镂空抽屉 (Autodesk Fusion 360 design; units mm, degrees)
part number: 2026-05-01-18-35-40-884
Autodesk Fusion 360 part; units mm, degrees
(part 1 of 2)
other "基础网格特征2"
other "修改1"
sketch "草图66" plane through (0, 0, 0) normal (0, 0, 1) x (1, 0, 0)
  line L0 (-100, -100) -> (100, -100)
  line L1 (100, -100) -> (100, 100)
  line L2 (100, 100) -> (-100, 100)
  line L3 (-100, 100) -> (-100, -100)
extrude "ex_drawer_body" add sketch "草图66" along normal blind 50
fillet "fillet_drawer_corners" radius 10 4 edges at (-100, 100, 25) (100, 100, 25) (100, -100, 25) (-100, -100, 25)
shell "shell_drawer" thickness 2 removed faces 1 at (30, -33.3333, 50)
sketch "草图68" plane through (0, -100, 0) normal (0, -1, 0) x (1, 0, 0)
  line L0 (-90, 50) -> (-90, 0)
  line L1 (-90, 0) -> (90, 0)
  line L2 (90, 0) -> (90, 50)
  line L3 (90, 50) -> (-90, 50)
  line L4 (-32.5, 44) -> (32.5, 44)
  line L5 (32.5, 29) -> (-32.5, 29)
  arc A0 (32.5, 29) -> (32.5, 44) centre (32.5, 36.5) ccw
  arc A1 (-32.5, 44) -> (-32.5, 29) centre (-32.5, 36.5) ccw
extrude "cut_grip_drawer" cut sketch "草图68" against normal blind 3 contours L4 L5 A0 A1
sketch "草图69" plane through (-100, 0, 0) normal (-1, 0, 0) x (0, -1, 0)
  line L0 (90, 0) -> (90, 50)
  line L1 (90, 50) -> (-90, 50)
  line L2 (-90, 50) -> (-90, 0)
  line L3 (-90, 0) -> (90, 0)
  line L4 (-81, 14) -> (-85.3301, 11.5)
  line L5 (-85.3301, 11.5) -> (-85.3301, 6.5)
  line L6 (-85.3301, 6.5) -> (-81, 4)
  line L7 (-81, 4) -> (-76.6699, 6.5)
  line L8 (-76.6699, 6.5) -> (-76.6699, 11.5)
  line L9 (-76.6699, 11.5) -> (-81, 14)
  line L10 (-70.3397, 14) -> (-74.6699, 11.5)
  line L11 (-74.6699, 11.5) -> (-74.6699, 6.5)
  line L12 (-74.6699, 6.5) -> (-70.3397, 4)
  line L13 (-70.3397, 4) -> (-66.0096, 6.5)
  line L14 (-66.0096, 6.5) -> (-66.0096, 11.5)
  line L15 (-66.0096, 11.5) -> (-70.3397, 14)
  line L16 (-59.6795, 14) -> (-64.0096, 11.5)
  line L17 (-64.0096, 11.5) -> (-64.0096, 6.5)
  line L18 (-64.0096, 6.5) -> (-59.6795, 4)
  line L19 (-59.6795, 4) -> (-55.3494, 6.5)
  line L20 (-55.3494, 6.5) -> (-55.3494, 11.5)
  line L21 (-55.3494, 11.5) -> (-59.6795, 14)
  line L22 (-49.0192, 14) -> (-53.3494, 11.5)
  line L23 (-53.3494, 11.5) -> (-53.3494, 6.5)
  line L24 (-53.3494, 6.5) -> (-49.0192, 4)
  line L25 (-49.0192, 4) -> (-44.6891, 6.5)
  line L26 (-44.6891, 6.5) -> (-44.6891, 11.5)
  line L27 (-44.6891, 11.5) -> (-49.0192, 14)
  line L28 (-38.359, 14) -> (-42.6891, 11.5)
  line L29 (-42.6891, 11.5) -> (-42.6891, 6.5)
  line L30 (-42.6891, 6.5) -> (-38.359, 4)
  line L31 (-38.359, 4) -> (-34.0289, 6.5)
  line L32 (-34.0289, 6.5) -> (-34.0289, 11.5)
  line L33 (-34.0289, 11.5) -> (-38.359, 14)
  line L34 (-27.6987, 14) -> (-32.0289, 11.5)
  line L35 (-32.0289, 11.5) -> (-32.0289, 6.5)
  line L36 (-32.0289, 6.5) -> (-27.6987, 4)
  line L37 (-27.6987, 4) -> (-23.3686, 6.5)
  line L38 (-23.3686, 6.5) -> (-23.3686, 11.5)
  line L39 (-23.3686, 11.5) -> (-27.6987, 14)
  line L40 (-17.0385, 14) -> (-21.3686, 11.5)
  line L41 (-21.3686, 11.5) -> (-21.3686, 6.5)
  line L42 (-21.3686, 6.5) -> (-17.0385, 4)
  line L43 (-17.0385, 4) -> (-12.7083, 6.5)
  line L44 (-12.7083, 6.5) -> (-12.7083, 11.5)
  line L45 (-12.7083, 11.5) -> (-17.0385, 14)
  line L46 (-6.3782, 14) -> (-10.7083, 11.5)
  line L47 (-10.7083, 11.5) -> (-10.7083, 6.5)
  line L48 (-10.7083, 6.5) -> (-6.3782, 4)
  line L49 (-6.3782, 4) -> (-2.0481, 6.5)
  line L50 (-2.0481, 6.5) -> (-2.0481, 11.5)
  line L51 (-2.0481, 11.5) -> (-6.3782, 14)
  line L52 (4.282, 14) -> (-0.0481, 11.5)
  line L53 (-0.0481, 11.5) -> (-0.0481, 6.5)
  line L54 (-0.0481, 6.5) -> (4.282, 4)
  line L55 (4.282, 4) -> (8.6122, 6.5)
  line L56 (8.6122, 6.5) -> (8.6122, 11.5)
  line L57 (8.6122, 11.5) -> (4.282, 14)
  line L58 (14.9423, 14) -> (10.6122, 11.5)
  line L59 (10.6122, 11.5) -> (10.6122, 6.5)
  line L60 (10.6122, 6.5) -> (14.9423, 4)
  line L61 (14.9423, 4) -> (19.2724, 6.5)
  line L62 (19.2724, 6.5) -> (19.2724, 11.5)
  line L63 (19.2724, 11.5) -> (14.9423, 14)
  line L64 (25.6025, 14) -> (21.2724, 11.5)
  line L65 (21.2724, 11.5) -> (21.2724, 6.5)
  line L66 (21.2724, 6.5) -> (25.6025, 4)
  line L67 (25.6025, 4) -> (29.9327, 6.5)
  line L68 (29.9327, 6.5) -> (29.9327, 11.5)
  line L69 (29.9327, 11.5) -> (25.6025, 14)
  line L70 (36.2628, 14) -> (31.9327, 11.5)
  line L71 (31.9327, 11.5) -> (31.9327, 6.5)
  line L72 (31.9327, 6.5) -> (36.2628, 4)
  line L73 (36.2628, 4) -> (40.5929, 6.5)
  line L74 (40.5929, 6.5) -> (40.5929, 11.5)
  line L75 (40.5929, 11.5) -> (36.2628, 14)
  line L76 (46.923, 14) -> (42.5929, 11.5)
  line L77 (42.5929, 11.5) -> (42.5929, 6.5)
  line L78 (42.5929, 6.5) -> (46.923, 4)
  line L79 (46.923, 4) -> (51.2532, 6.5)
  line L80 (51.2532, 6.5) -> (51.2532, 11.5)
  line L81 (51.2532, 11.5) -> (46.923, 14)
  line L82 (57.5833, 14) -> (53.2532, 11.5)
  line L83 (53.2532, 11.5) -> (53.2532, 6.5)
  line L84 (53.2532, 6.5) -> (57.5833, 4)
  line L85 (57.5833, 4) -> (61.9134, 6.5)
  line L86 (61.9134, 6.5) -> (61.9134, 11.5)
  line L87 (61.9134, 11.5) -> (57.5833, 14)
  line L88 (68.2436, 14) -> (63.9134, 11.5)
  line L89 (63.9134, 11.5) -> (63.9134, 6.5)
  line L90 (63.9134, 6.5) -> (68.2436, 4)
  line L91 (68.2436, 4) -> (72.5737, 6.5)
  line L92 (72.5737, 6.5) -> (72.5737, 11.5)
  line L93 (72.5737, 11.5) -> (68.2436, 14)
  line L94 (78.9038, 14) -> (74.5737, 11.5)
  line L95 (74.5737, 11.5) -> (74.5737, 6.5)
  line L96 (74.5737, 6.5) -> (78.9038, 4)
  line L97 (78.9038, 4) -> (83.2339, 6.5)
  line L98 (83.2339, 6.5) -> (83.2339, 11.5)
  line L99 (83.2339, 11.5) -> (78.9038, 14)
  line L100 (-75.6699, 23.2321) -> (-80, 20.7321)
  line L101 (-80, 20.7321) -> (-80, 15.7321)
  line L102 (-80, 15.7321) -> (-75.6699, 13.2321)
  line L103 (-75.6699, 13.2321) -> (-71.3397, 15.7321)
  line L104 (-71.3397, 15.7321) -> (-71.3397, 20.7321)
  line L105 (-71.3397, 20.7321) -> (-75.6699, 23.2321)
  line L106 (-65.0096, 23.2321) -> (-69.3397, 20.7321)
  line L107 (-69.3397, 20.7321) -> (-69.3397, 15.7321)
  line L108 (-69.3397, 15.7321) -> (-65.0096, 13.2321)
  line L109 (-65.0096, 13.2321) -> (-60.6795, 15.7321)
  line L110 (-60.6795, 15.7321) -> (-60.6795, 20.7321)
  line L111 (-60.6795, 20.7321) -> (-65.0096, 23.2321)
  line L112 (-54.3494, 23.2321) -> (-58.6795, 20.7321)
  line L113 (-58.6795, 20.7321) -> (-58.6795, 15.7321)
  line L114 (-58.6795, 15.7321) -> (-54.3494, 13.2321)
  line L115 (-54.3494, 13.2321) -> (-50.0192, 15.7321)
  line L116 (-50.0192, 15.7321) -> (-50.0192, 20.7321)
  line L117 (-50.0192, 20.7321) -> (-54.3494, 23.2321)
  line L118 (-43.6891, 23.2321) -> (-48.0192, 20.7321)
  line L119 (-48.0192, 20.7321) -> (-48.0192, 15.7321)
  line L120 (-48.0192, 15.7321) -> (-43.6891, 13.2321)
  line L121 (-43.6891, 13.2321) -> (-39.359, 15.7321)
  line L122 (-39.359, 15.7321) -> (-39.359, 20.7321)
  line L123 (-39.359, 20.7321) -> (-43.6891, 23.2321)
  line L124 (-33.0289, 23.2321) -> (-37.359, 20.7321)
  line L125 (-37.359, 20.7321) -> (-37.359, 15.7321)
  line L126 (-37.359, 15.7321) -> (-33.0289, 13.2321)
  line L127 (-33.0289, 13.2321) -> (-28.6987, 15.7321)
  line L128 (-28.6987, 15.7321) -> (-28.6987, 20.7321)
  line L129 (-28.6987, 20.7321) -> (-33.0289, 23.2321)
  line L130 (-22.3686, 23.2321) -> (-26.6987, 20.7321)
  line L131 (-26.6987, 20.7321) -> (-26.6987, 15.7321)
  line L132 (-26.6987, 15.7321) -> (-22.3686, 13.2321)
  line L133 (-22.3686, 13.2321) -> (-18.0385, 15.7321)
  line L134 (-18.0385, 15.7321) -> (-18.0385, 20.7321)
  line L135 (-18.0385, 20.7321) -> (-22.3686, 23.2321)
  line L136 (-11.7083, 23.2321) -> (-16.0385, 20.7321)
  line L137 (-16.0385, 20.7321) -> (-16.0385, 15.7321)
  line L138 (-16.0385, 15.7321) -> (-11.7083, 13.2321)
  line L139 (-11.7083, 13.2321) -> (-7.3782, 15.7321)
  line L140 (-7.3782, 15.7321) -> (-7.3782, 20.7321)
  line L141 (-7.3782, 20.7321) -> (-11.7083, 23.2321)
  line L142 (-1.0481, 23.2321) -> (-5.3782, 20.7321)
  line L143 (-5.3782, 20.7321) -> (-5.3782, 15.7321)
  line L144 (-5.3782, 15.7321) -> (-1.0481, 13.2321)
  line L145 (-1.0481, 13.2321) -> (3.282, 15.7321)
  line L146 (3.282, 15.7321) -> (3.282, 20.7321)
  line L147 (3.282, 20.7321) -> (-1.0481, 23.2321)
  line L148 (9.6122, 23.2321) -> (5.282, 20.7321)
  line L149 (5.282, 20.7321) -> (5.282, 15.7321)
  line L150 (5.282, 15.7321) -> (9.6122, 13.2321)
  line L151 (9.6122, 13.2321) -> (13.9423, 15.7321)
  line L152 (13.9423, 15.7321) -> (13.9423, 20.7321)
  line L153 (13.9423, 20.7321) -> (9.6122, 23.2321)
  line L154 (20.2724, 23.2321) -> (15.9423, 20.7321)
  line L155 (15.9423, 20.7321) -> (15.9423, 15.7321)
  line L156 (15.9423, 15.7321) -> (20.2724, 13.2321)
  line L157 (20.2724, 13.2321) -> (24.6025, 15.7321)
  line L158 (24.6025, 15.7321) -> (24.6025, 20.7321)
  line L159 (24.6025, 20.7321) -> (20.2724, 23.2321)
  line L160 (30.9327, 23.2321) -> (26.6025, 20.7321)
  line L161 (26.6025, 20.7321) -> (26.6025, 15.7321)
  line L162 (26.6025, 15.7321) -> (30.9327, 13.2321)
  line L163 (30.9327, 13.2321) -> (35.2628, 15.7321)
  line L164 (35.2628, 15.7321) -> (35.2628, 20.7321)
  line L165 (35.2628, 20.7321) -> (30.9327, 23.2321)
  line L166 (41.5929, 23.2321) -> (37.2628, 20.7321)
  line L167 (37.2628, 20.7321) -> (37.2628, 15.7321)
  line L168 (37.2628, 15.7321) -> (41.5929, 13.2321)
  line L169 (41.5929, 13.2321) -> (45.923, 15.7321)
  line L170 (45.923, 15.7321) -> (45.923, 20.7321)
  line L171 (45.923, 20.7321) -> (41.5929, 23.2321)
  line L172 (52.2532, 23.2321) -> (47.923, 20.7321)
  line L173 (47.923, 20.7321) -> (47.923, 15.7321)
  line L174 (47.923, 15.7321) -> (52.2532, 13.2321)
  line L175 (52.2532, 13.2321) -> (56.5833, 15.7321)
  line L176 (56.5833, 15.7321) -> (56.5833, 20.7321)
  line L177 (56.5833, 20.7321) -> (52.2532, 23.2321)
  line L178 (62.9134, 23.2321) -> (58.5833, 20.7321)
  line L179 (58.5833, 20.7321) -> (58.5833, 15.7321)
  line L180 (58.5833, 15.7321) -> (62.9134, 13.2321)
  line L181 (62.9134, 13.2321) -> (67.2436, 15.7321)
  line L182 (67.2436, 15.7321) -> (67.2436, 20.7321)
  line L183 (67.2436, 20.7321) -> (62.9134, 23.2321)
  line L184 (73.5737, 23.2321) -> (69.2436, 20.7321)
  line L185 (69.2436, 20.7321) -> (69.2436, 15.7321)
  line L186 (69.2436, 15.7321) -> (73.5737, 13.2321)
  line L187 (73.5737, 13.2321) -> (77.9038, 15.7321)
  line L188 (77.9038, 15.7321) -> (77.9038, 20.7321)
  line L189 (77.9038, 20.7321) -> (73.5737, 23.2321)
  line L190 (-81, 32.4641) -> (-85.3301, 29.9641)
  line L191 (-85.3301, 29.9641) -> (-85.3301, 24.9641)
  line L192 (-85.3301, 24.9641) -> (-81, 22.4641)
  line L193 (-81, 22.4641) -> (-76.6699, 24.9641)
  line L194 (-76.6699, 24.9641) -> (-76.6699, 29.9641)
  line L195 (-76.6699, 29.9641) -> (-81, 32.4641)
  line L196 (-70.3397, 32.4641) -> (-74.6699, 29.9641)
  line L197 (-74.6699, 29.9641) -> (-74.6699, 24.9641)
  line L198 (-74.6699, 24.9641) -> (-70.3397, 22.4641)
  line L199 (-70.3397, 22.4641) -> (-66.0096, 24.9641)
  line L200 (-66.0096, 24.9641) -> (-66.0096, 29.9641)
  line L201 (-66.0096, 29.9641) -> (-70.3397, 32.4641)
  line L202 (-59.6795, 32.4641) -> (-64.0096, 29.9641)
  line L203 (-64.0096, 29.9641) -> (-64.0096, 24.9641)
  line L204 (-64.0096, 24.9641) -> (-59.6795, 22.4641)
  line L205 (-59.6795, 22.4641) -> (-55.3494, 24.9641)
  line L206 (-55.3494, 24.9641) -> (-55.3494, 29.9641)
  line L207 (-55.3494, 29.9641) -> (-59.6795, 32.4641)
  line L208 (-49.0192, 32.4641) -> (-53.3494, 29.9641)
  line L209 (-53.3494, 29.9641) -> (-53.3494, 24.9641)
  line L210 (-53.3494, 24.9641) -> (-49.0192, 22.4641)
  line L211 (-49.0192, 22.4641) -> (-44.6891, 24.9641)
  line L212 (-44.6891, 24.9641) -> (-44.6891, 29.9641)
  line L213 (-44.6891, 29.9641) -> (-49.0192, 32.4641)
  line L214 (-38.359, 32.4641) -> (-42.6891, 29.9641)
  line L215 (-42.6891, 29.9641) -> (-42.6891, 24.9641)
  line L216 (-42.6891, 24.9641) -> (-38.359, 22.4641)
  line L217 (-38.359, 22.4641) -> (-34.0289, 24.9641)
  line L218 (-34.0289, 24.9641) -> (-34.0289, 29.9641)
  line L219 (-34.0289, 29.9641) -> (-38.359, 32.4641)
  line L220 (-27.6987, 32.4641) -> (-32.0289, 29.9641)
  line L221 (-32.0289, 29.9641) -> (-32.0289, 24.9641)
  line L222 (-32.0289, 24.9641) -> (-27.6987, 22.4641)
  line L223 (-27.6987, 22.4641) -> (-23.3686, 24.9641)
  line L224 (-23.3686, 24.9641) -> (-23.3686, 29.9641)
  line L225 (-23.3686, 29.9641) -> (-27.6987, 32.4641)
  line L226 (-17.0385, 32.4641) -> (-21.3686, 29.9641)
  line L227 (-21.3686, 29.9641) -> (-21.3686, 24.9641)
  line L228 (-21.3686, 24.9641) -> (-17.0385, 22.4641)
  line L229 (-17.0385, 22.4641) -> (-12.7083, 24.9641)
  line L230 (-12.7083, 24.9641) -> (-12.7083, 29.9641)
  line L231 (-12.7083, 29.9641) -> (-17.0385, 32.4641)
  line L232 (-6.3782, 32.4641) -> (-10.7083, 29.9641)
  line L233 (-10.7083, 29.9641) -> (-10.7083, 24.9641)
  line L234 (-10.7083, 24.9641) -> (-6.3782, 22.4641)
  line L235 (-6.3782, 22.4641) -> (-2.0481, 24.9641)
  line L236 (-2.0481, 24.9641) -> (-2.0481, 29.9641)
  line L237 (-2.0481, 29.9641) -> (-6.3782, 32.4641)
  line L238 (4.282, 32.4641) -> (-0.0481, 29.9641)
  line L239 (-0.0481, 29.9641) -> (-0.0481, 24.9641)
  line L240 (-0.0481, 24.9641) -> (4.282, 22.4641)
  line L241 (4.282, 22.4641) -> (8.6122, 24.9641)
  line L242 (8.6122, 24.9641) -> (8.6122, 29.9641)
  line L243 (8.6122, 29.9641) -> (4.282, 32.4641)
  line L244 (14.9423, 32.4641) -> (10.6122, 29.9641)
  line L245 (10.6122, 29.9641) -> (10.6122, 24.9641)
  line L246 (10.6122, 24.9641) -> (14.9423, 22.4641)
  line L247 (14.9423, 22.4641) -> (19.2724, 24.9641)
  line L248 (19.2724, 24.9641) -> (19.2724, 29.9641)
  line L249 (19.2724, 29.9641) -> (14.9423, 32.4641)
  line L250 (25.6025, 32.4641) -> (21.2724, 29.9641)
  line L251 (21.2724, 29.9641) -> (21.2724, 24.9641)
  line L252 (21.2724, 24.9641) -> (25.6025, 22.4641)
  line L253 (25.6025, 22.4641) -> (29.9327, 24.9641)
  line L254 (29.9327, 24.9641) -> (29.9327, 29.9641)
  line L255 (29.9327, 29.9641) -> (25.6025, 32.4641)
  line L256 (36.2628, 32.4641) -> (31.9327, 29.9641)
  line L257 (31.9327, 29.9641) -> (31.9327, 24.9641)
  line L258 (31.9327, 24.9641) -> (36.2628, 22.4641)
  line L259 (36.2628, 22.4641) -> (40.5929, 24.9641)
  line L260 (40.5929, 24.9641) -> (40.5929, 29.9641)
  line L261 (40.5929, 29.9641) -> (36.2628, 32.4641)
  line L262 (46.923, 32.4641) -> (42.5929, 29.9641)
  line L263 (42.5929, 29.9641) -> (42.5929, 24.9641)
  line L264 (42.5929, 24.9641) -> (46.923, 22.4641)
  line L265 (46.923, 22.4641) -> (51.2532, 24.9641)
  line L266 (51.2532, 24.9641) -> (51.2532, 29.9641)
  line L267 (51.2532, 29.9641) -> (46.923, 32.4641)
  line L268 (57.5833, 32.4641) -> (53.2532, 29.9641)
  line L269 (53.2532, 29.9641) -> (53.2532, 24.9641)
  line L270 (53.2532, 24.9641) -> (57.5833, 22.4641)
  line L271 (57.5833, 22.4641) -> (61.9134, 24.9641)
  line L272 (61.9134, 24.9641) -> (61.9134, 29.9641)
  line L273 (61.9134, 29.9641) -> (57.5833, 32.4641)
  line L274 (68.2436, 32.4641) -> (63.9134, 29.9641)
  line L275 (63.9134, 29.9641) -> (63.9134, 24.9641)
  line L276 (63.9134, 24.9641) -> (68.2436, 22.4641)
  line L277 (68.2436, 22.4641) -> (72.5737, 24.9641)
  line L278 (72.5737, 24.9641) -> (72.5737, 29.9641)
  line L279 (72.5737, 29.9641) -> (68.2436, 32.4641)
  line L280 (78.9038, 32.4641) -> (74.5737, 29.9641)
  line L281 (74.5737, 29.9641) -> (74.5737, 24.9641)
  line L282 (74.5737, 24.9641) -> (78.9038, 22.4641)
  line L283 (78.9038, 22.4641) -> (83.2339, 24.9641)
  line L284 (83.2339, 24.9641) -> (83.2339, 29.9641)
  line L285 (83.2339, 29.9641) -> (78.9038, 32.4641)
  line L286 (-75.6699, 41.6962) -> (-80, 39.1962)
  line L287 (-80, 39.1962) -> (-80, 34.1962)
  line L288 (-80, 34.1962) -> (-75.6699, 31.6962)
  line L289 (-75.6699, 31.6962) -> (-71.3397, 34.1962)
  line L290 (-71.3397, 34.1962) -> (-71.3397, 39.1962)
  line L291 (-71.3397, 39.1962) -> (-75.6699, 41.6962)
  line L292 (-65.0096, 41.6962) -> (-69.3397, 39.1962)
  line L293 (-69.3397, 39.1962) -> (-69.3397, 34.1962)
  line L294 (-69.3397, 34.1962) -> (-65.0096, 31.6962)
  line L295 (-65.0096, 31.6962) -> (-60.6795, 34.1962)
  line L296 (-60.6795, 34.1962) -> (-60.6795, 39.1962)
  line L297 (-60.6795, 39.1962) -> (-65.0096, 41.6962)
  line L298 (-54.3494, 41.6962) -> (-58.6795, 39.1962)
  line L299 (-58.6795, 39.1962) -> (-58.6795, 34.1962)
  line L300 (-58.6795, 34.1962) -> (-54.3494, 31.6962)
  line L301 (-54.3494, 31.6962) -> (-50.0192, 34.1962)
  line L302 (-50.0192, 34.1962) -> (-50.0192, 39.1962)
  line L303 (-50.0192, 39.1962) -> (-54.3494, 41.6962)
  line L304 (-43.6891, 41.6962) -> (-48.0192, 39.1962)
  line L305 (-48.0192, 39.1962) -> (-48.0192, 34.1962)
  line L306 (-48.0192, 34.1962) -> (-43.6891, 31.6962)
  line L307 (-43.6891, 31.6962) -> (-39.359, 34.1962)
  line L308 (-39.359, 34.1962) -> (-39.359, 39.1962)
  line L309 (-39.359, 39.1962) -> (-43.6891, 41.6962)
  line L310 (-33.0289, 41.6962) -> (-37.359, 39.1962)
  line L311 (-37.359, 39.1962) -> (-37.359, 34.1962)
  line L312 (-37.359, 34.1962) -> (-33.0289, 31.6962)
  line L313 (-33.0289, 31.6962) -> (-28.6987, 34.1962)
  line L314 (-28.6987, 34.1962) -> (-28.6987, 39.1962)
  line L315 (-28.6987, 39.1962) -> (-33.0289, 41.6962)
  line L316 (-22.3686, 41.6962) -> (-26.6987, 39.1962)
  line L317 (-26.6987, 39.1962) -> (-26.6987, 34.1962)
  line L318 (-26.6987, 34.1962) -> (-22.3686, 31.6962)
  line L319 (-22.3686, 31.6962) -> (-18.0385, 34.1962)
  line L320 (-18.0385, 34.1962) -> (-18.0385, 39.1962)
  line L321 (-18.0385, 39.1962) -> (-22.3686, 41.6962)
  line L322 (-11.7083, 41.6962) -> (-16.0385, 39.1962)
  line L323 (-16.0385, 39.1962) -> (-16.0385, 34.1962)
  line L324 (-16.0385, 34.1962) -> (-11.7083, 31.6962)
  line L325 (-11.7083, 31.6962) -> (-7.3782, 34.1962)
  line L326 (-7.3782, 34.1962) -> (-7.3782, 39.1962)
  line L327 (-7.3782, 39.1962) -> (-11.7083, 41.6962)
  line L328 (-1.0481, 41.6962) -> (-5.3782, 39.1962)
  line L329 (-5.3782, 39.1962) -> (-5.3782, 34.1962)
  line L330 (-5.3782, 34.1962) -> (-1.0481, 31.6962)
  line L331 (-1.0481, 31.6962) -> (3.282, 34.1962)
  line L332 (3.282, 34.1962) -> (3.282, 39.1962)
  line L333 (3.282, 39.1962) -> (-1.0481, 41.6962)
  line L334 (9.6122, 41.6962) -> (5.282, 39.1962)
  line L335 (5.282, 39.1962) -> (5.282, 34.1962)
  line L336 (5.282, 34.1962) -> (9.6122, 31.6962)
  line L337 (9.6122, 31.6962) -> (13.9423, 34.1962)
  line L338 (13.9423, 34.1962) -> (13.9423, 39.1962)
  line L339 (13.9423, 39.1962) -> (9.6122, 41.6962)
  line L340 (20.2724, 41.6962) -> (15.9423, 39.1962)
  line L341 (15.9423, 39.1962) -> (15.9423, 34.1962)
  line L342 (15.9423, 34.1962) -> (20.2724, 31.6962)
  line L343 (20.2724, 31.6962) -> (24.6025, 34.1962)
  line L344 (24.6025, 34.1962) -> (24.6025, 39.1962)
  line L345 (24.6025, 39.1962) -> (20.2724, 41.6962)
  line L346 (30.9327, 41.6962) -> (26.6025, 39.1962)
  line L347 (26.6025, 39.1962) -> (26.6025, 34.1962)
  line L348 (26.6025, 34.1962) -> (30.9327, 31.6962)
  line L349 (30.9327, 31.6962) -> (35.2628, 34.1962)
  line L350 (35.2628, 34.1962) -> (35.2628, 39.1962)
  line L351 (35.2628, 39.1962) -> (30.9327, 41.6962)
  line L352 (41.5929, 41.6962) -> (37.2628, 39.1962)
  line L353 (37.2628, 39.1962) -> (37.2628, 34.1962)
  line L354 (37.2628, 34.1962) -> (41.5929, 31.6962)
  line L355 (41.5929, 31.6962) -> (45.923, 34.1962)
  line L356 (45.923, 34.1962) -> (45.923, 39.1962)
  line L357 (45.923, 39.1962) -> (41.5929, 41.6962)
  line L358 (52.2532, 41.6962) -> (47.923, 39.1962)
  line L359 (47.923, 39.1962) -> (47.923, 34.1962)
  line L360 (47.923, 34.1962) -> (52.2532, 31.6962)
  line L361 (52.2532, 31.6962) -> (56.5833, 34.1962)
  line L362 (56.5833, 34.1962) -> (56.5833, 39.1962)
  line L363 (56.5833, 39.1962) -> (52.2532, 41.6962)
  line L364 (62.9134, 41.6962) -> (58.5833, 39.1962)
  line L365 (58.5833, 39.1962) -> (58.5833, 34.1962)
  line L366 (58.5833, 34.1962) -> (62.9134, 31.6962)
  line L367 (62.9134, 31.6962) -> (67.2436, 34.1962)
  line L368 (67.2436, 34.1962) -> (67.2436, 39.1962)
  line L369 (67.2436, 39.1962) -> (62.9134, 41.6962)
  line L370 (73.5737, 41.6962) -> (69.2436, 39.1962)
  line L371 (69.2436, 39.1962) -> (69.2436, 34.1962)
  line L372 (69.2436, 34.1962) -> (73.5737, 31.6962)
  line L373 (73.5737, 31.6962) -> (77.9038, 34.1962)
  line L374 (77.9038, 34.1962) -> (77.9038, 39.1962)
  line L375 (77.9038, 39.1962) -> (73.5737, 41.6962)
extrude "cut_hex_drawer_left" cut sketch "草图69" against normal blind 3 contours L4 L5 L6 L7 L8 L9 | L10 L11 L12 L13 L14 L15 | L16 L17 L18 L19 L20 L21 | L22 L23 L24 L25 L26 L27 | L28 L29 L30 L31 L32 L33 | L34 L35 L36 L37 L38 L39 | L40 L41 L42 L43 L44 L45 | L46 L47 L48 L49 L50 L51 | L52 L53 L54 L55 L56 L57 | L58 L59 L60 L61 L62 L63 | L64 L65 L66 L67 L68 L69 | L70 L71 L72 L73 L74 L75 | L76 L77 L78 L79 L80 L81 | L82 L83 L84 L85 L86 L87 | L88 L89 L90 L91 L92 L93 | L94 L95 L96 L97 L98 L99 | L100 L101 L102 L103 L104 L105 | L106 L107 L108 L109 L110 L111 | L112 L113 L114 L115 L116 L117 | L118 L119 L120 L121 L122 L123 | L124 L125 L126 L127 L128 L129 | L130 L131 L132 L133 L134 L135 | L136 L137 L138 L139 L140 L141 | L142 L143 L144 L145 L146 L147 | L148 L149 L150 L151 L152 L153 | L154 L155 L156 L157 L158 L159 | L160 L161 L162 L163 L164 L165 | L166 L167 L168 L169 L170 L171 | L172 L173 L174 L175 L176 L177 | L178 L179 L180 L181 L182 L183 | L184 L185 L186 L187 L188 L189 | L190 L191 L192 L193 L194 L195 | L196 L197 L198 L199 L200 L201 | L202 L203 L204 L205 L206 L207 | L208 L209 L210 L211 L212 L213 | L214 L215 L216 L217 L218 L219 | L220 L221 L222 L223 L224 L225 | L226 L227 L228 L229 L230 L231 | L232 L233 L234 L235 L236 L237 | L238 L239 L240 L241 L242 L243 | L244 L245 L246 L247 L248 L249 | L250 L251 L252 L253 L254 L255 | L256 L257 L258 L259 L260 L261 | L262 L263 L264 L265 L266 L267 | L268 L269 L270 L271 L272 L273 | L274 L275 L276 L277 L278 L279 | L280 L281 L282 L283 L284 L285 | L286 L287 L288 L289 L290 L291 | L292 L293 L294 L295 L296 L297 | L298 L299 L300 L301 L302 L303 | L304 L305 L306 L307 L308 L309 | L310 L311 L312 L313 L314 L315 | L316 L317 L318 L319 L320 L321 | L322 L323 L324 L325 L326 L327 | L328 L329 L330 L331 L332 L333 | L334 L335 L336 L337 L338 L339 | L340 L341 L342 L343 L344 L345 | L346 L347 L348 L349 L350 L351 | L352 L353 L354 L355 L356 L357 | L358 L359 L360 L361 L362 L363 | L364 L365 L366 L367 L368 L369 | L370 L371 L372 L373 L374 L375
sketch "草图70" plane through (100, 0, 0) normal (1, 0, 0) x (0, 1, 0)
  line L0 (-90, 50) -> (-90, 0)
  line L1 (-90, 0) -> (90, 0)
  line L2 (90, 0) -> (90, 50)
  line L3 (90, 50) -> (-90, 50)
  line L4 (-81, 14) -> (-85.3301, 11.5)
  line L5 (-85.3301, 11.5) -> (-85.3301, 6.5)
  line L6 (-85.3301, 6.5) -> (-81, 4)
  line L7 (-81, 4) -> (-76.6699, 6.5)
  line L8 (-76.6699, 6.5) -> (-76.6699, 11.5)
  line L9 (-76.6699, 11.5) -> (-81, 14)
  line L10 (-70.3397, 14) -> (-74.6699, 11.5)
  line L11 (-74.6699, 11.5) -> (-74.6699, 6.5)
  line L12 (-74.6699, 6.5) -> (-70.3397, 4)
  line L13 (-70.3397, 4) -> (-66.0096, 6.5)
  line L14 (-66.0096, 6.5) -> (-66.0096, 11.5)
  line L15 (-66.0096, 11.5) -> (-70.3397, 14)
  line L16 (-59.6795, 14) -> (-64.0096, 11.5)
  line L17 (-64.0096, 11.5) -> (-64.0096, 6.5)
  line L18 (-64.0096, 6.5) -> (-59.6795, 4)
  line L19 (-59.6795, 4) -> (-55.3494, 6.5)
  line L20 (-55.3494, 6.5) -> (-55.3494, 11.5)
  line L21 (-55.3494, 11.5) -> (-59.6795, 14)
  line L22 (-49.0192, 14) -> (-53.3494, 11.5)
  line L23 (-53.3494, 11.5) -> (-53.3494, 6.5)
  line L24 (-53.3494, 6.5) -> (-49.0192, 4)
  line L25 (-49.0192, 4) -> (-44.6891, 6.5)
  line L26 (-44.6891, 6.5) -> (-44.6891, 11.5)
  line L27 (-44.6891, 11.5) -> (-49.0192, 14)
  line L28 (-38.359, 14) -> (-42.6891, 11.5)
  line L29 (-42.6891, 11.5) -> (-42.6891, 6.5)
  line L30 (-42.6891, 6.5) -> (-38.359, 4)
  line L31 (-38.359, 4) -> (-34.0289, 6.5)
  line L32 (-34.0289, 6.5) -> (-34.0289, 11.5)
  line L33 (-34.0289, 11.5) -> (-38.359, 14)
  line L34 (-27.6987, 14) -> (-32.0289, 11.5)
  line L35 (-32.0289, 11.5) -> (-32.0289, 6.5)
  line L36 (-32.0289, 6.5) -> (-27.6987, 4)
  line L37 (-27.6987, 4) -> (-23.3686, 6.5)
  line L38 (-23.3686, 6.5) -> (-23.3686, 11.5)
  line L39 (-23.3686, 11.5) -> (-27.6987, 14)
  line L40 (-17.0385, 14) -> (-21.3686, 11.5)
  line L41 (-21.3686, 11.5) -> (-21.3686, 6.5)
  line L42 (-21.3686, 6.5) -> (-17.0385, 4)
  line L43 (-17.0385, 4) -> (-12.7083, 6.5)
  line L44 (-12.7083, 6.5) -> (-12.7083, 11.5)
  line L45 (-12.7083, 11.5) -> (-17.0385, 14)
  line L46 (-6.3782, 14) -> (-10.7083, 11.5)
  line L47 (-10.7083, 11.5) -> (-10.7083, 6.5)
  line L48 (-10.7083, 6.5) -> (-6.3782, 4)
  line L49 (-6.3782, 4) -> (-2.0481, 6.5)
  line L50 (-2.0481, 6.5) -> (-2.0481, 11.5)
  line L51 (-2.0481, 11.5) -> (-6.3782, 14)
  line L52 (4.282, 14) -> (-0.0481, 11.5)
  line L53 (-0.0481, 11.5) -> (-0.0481, 6.5)
  line L54 (-0.0481, 6.5) -> (4.282, 4)
  line L55 (4.282, 4) -> (8.6122, 6.5)
  line L56 (8.6122, 6.5) -> (8.6122, 11.5)
  line L57 (8.6122, 11.5) -> (4.282, 14)
  line L58 (14.9423, 14) -> (10.6122, 11.5)
  line L59 (10.6122, 11.5) -> (10.6122, 6.5)
  line L60 (10.6122, 6.5) -> (14.9423, 4)
  line L61 (14.9423, 4) -> (19.2724, 6.5)
  line L62 (19.2724, 6.5) -> (19.2724, 11.5)
  line L63 (19.2724, 11.5) -> (14.9423, 14)
  line L64 (25.6025, 14) -> (21.2724, 11.5)
  line L65 (21.2724, 11.5) -> (21.2724, 6.5)
  line L66 (21.2724, 6.5) -> (25.6025, 4)
  line L67 (25.6025, 4) -> (29.9327, 6.5)
  line L68 (29.9327, 6.5) -> (29.9327, 11.5)
  line L69 (29.9327, 11.5) -> (25.6025, 14)
  line L70 (36.2628, 14) -> (31.9327, 11.5)
  line L71 (31.9327, 11.5) -> (31.9327, 6.5)
  line L72 (31.9327, 6.5) -> (36.2628, 4)
  line L73 (36.2628, 4) -> (40.5929, 6.5)
  line L74 (40.5929, 6.5) -> (40.5929, 11.5)
  line L75 (40.5929, 11.5) -> (36.2628, 14)
  line L76 (46.923, 14) -> (42.5929, 11.5)
  line L77 (42.5929, 11.5) -> (42.5929, 6.5)
  line L78 (42.5929, 6.5) -> (46.923, 4)
  line L79 (46.923, 4) -> (51.2532, 6.5)
  line L80 (51.2532, 6.5) -> (51.2532, 11.5)
  line L81 (51.2532, 11.5) -> (46.923, 14)
  line L82 (57.5833, 14) -> (53.2532, 11.5)
  line L83 (53.2532, 11.5) -> (53.2532, 6.5)
  line L84 (53.2532, 6.5) -> (57.5833, 4)
  line L85 (57.5833, 4) -> (61.9134, 6.5)
  line L86 (61.9134, 6.5) -> (61.9134, 11.5)
  line L87 (61.9134, 11.5) -> (57.5833, 14)
  line L88 (68.2436, 14) -> (63.9134, 11.5)
  line L89 (63.9134, 11.5) -> (63.9134, 6.5)
  line L90 (63.9134, 6.5) -> (68.2436, 4)
  line L91 (68.2436, 4) -> (72.5737, 6.5)
  line L92 (72.5737, 6.5) -> (72.5737, 11.5)
  line L93 (72.5737, 11.5) -> (68.2436, 14)
  line L94 (78.9038, 14) -> (74.5737, 11.5)
  line L95 (74.5737, 11.5) -> (74.5737, 6.5)
  line L96 (74.5737, 6.5) -> (78.9038, 4)
  line L97 (78.9038, 4) -> (83.2339, 6.5)
  line L98 (83.2339, 6.5) -> (83.2339, 11.5)
  line L99 (83.2339, 11.5) -> (78.9038, 14)
  line L100 (-75.6699, 23.2321) -> (-80, 20.7321)
  line L101 (-80, 20.7321) -> (-80, 15.7321)
  line L102 (-80, 15.7321) -> (-75.6699, 13.2321)
  line L103 (-75.6699, 13.2321) -> (-71.3397, 15.7321)
  line L104 (-71.3397, 15.7321) -> (-71.3397, 20.7321)
  line L105 (-71.3397, 20.7321) -> (-75.6699, 23.2321)
  line L106 (-65.0096, 23.2321) -> (-69.3397, 20.7321)
  line L107 (-69.3397, 20.7321) -> (-69.3397, 15.7321)
  line L108 (-69.3397, 15.7321) -> (-65.0096, 13.2321)
  line L109 (-65.0096, 13.2321) -> (-60.6795, 15.7321)
  line L110 (-60.6795, 15.7321) -> (-60.6795, 20.7321)
  line L111 (-60.6795, 20.7321) -> (-65.0096, 23.2321)
  line L112 (-54.3494, 23.2321) -> (-58.6795, 20.7321)
  line L113 (-58.6795, 20.7321) -> (-58.6795, 15.7321)
  line L114 (-58.6795, 15.7321) -> (-54.3494, 13.2321)
  line L115 (-54.3494, 13.2321) -> (-50.0192, 15.7321)
  line L116 (-50.0192, 15.7321) -> (-50.0192, 20.7321)
  line L117 (-50.0192, 20.7321) -> (-54.3494, 23.2321)
  line L118 (-43.6891, 23.2321) -> (-48.0192, 20.7321)
  line L119 (-48.0192, 20.7321) -> (-48.0192, 15.7321)
  line L120 (-48.0192, 15.7321) -> (-43.6891, 13.2321)
  line L121 (-43.6891, 13.2321) -> (-39.359, 15.7321)
  line L122 (-39.359, 15.7321) -> (-39.359, 20.7321)
  line L123 (-39.359, 20.7321) -> (-43.6891, 23.2321)
  line L124 (-33.0289, 23.2321) -> (-37.359, 20.7321)
  line L125 (-37.359, 20.7321) -> (-37.359, 15.7321)
  line L126 (-37.359, 15.7321) -> (-33.0289, 13.2321)
  line L127 (-33.0289, 13.2321) -> (-28.6987, 15.7321)
  line L128 (-28.6987, 15.7321) -> (-28.6987, 20.7321)
  line L129 (-28.6987, 20.7321) -> (-33.0289, 23.2321)
  line L130 (-22.3686, 23.2321) -> (-26.6987, 20.7321)
  line L131 (-26.6987, 20.7321) -> (-26.6987, 15.7321)
  line L132 (-26.6987, 15.7321) -> (-22.3686, 13.2321)
  line L133 (-22.3686, 13.2321) -> (-18.0385, 15.7321)
  line L134 (-18.0385, 15.7321) -> (-18.0385, 20.7321)
  line L135 (-18.0385, 20.7321) -> (-22.3686, 23.2321)
  line L136 (-11.7083, 23.2321) -> (-16.0385, 20.7321)
  line L137 (-16.0385, 20.7321) -> (-16.0385, 15.7321)
  line L138 (-16.0385, 15.7321) -> (-11.7083, 13.2321)
  line L139 (-11.7083, 13.2321) -> (-7.3782, 15.7321)
  line L140 (-7.3782, 15.7321) -> (-7.3782, 20.7321)
  line L141 (-7.3782, 20.7321) -> (-11.7083, 23.2321)
  line L142 (-1.0481, 23.2321) -> (-5.3782, 20.7321)
  line L143 (-5.3782, 20.7321) -> (-5.3782, 15.7321)
  line L144 (-5.3782, 15.7321) -> (-1.0481, 13.2321)
  line L145 (-1.0481, 13.2321) -> (3.282, 15.7321)
  line L146 (3.282, 15.7321) -> (3.282, 20.7321)
  line L147 (3.282, 20.7321) -> (-1.0481, 23.2321)
  line L148 (9.6122, 23.2321) -> (5.282, 20.7321)
  line L149 (5.282, 20.7321) -> (5.282, 15.7321)
  line L150 (5.282, 15.7321) -> (9.6122, 13.2321)
  line L151 (9.6122, 13.2321) -> (13.9423, 15.7321)
  line L152 (13.9423, 15.7321) -> (13.9423, 20.7321)
  line L153 (13.9423, 20.7321) -> (9.6122, 23.2321)
  line L154 (20.2724, 23.2321) -> (15.9423, 20.7321)
  line L155 (15.9423, 20.7321) -> (15.9423, 15.7321)
  line L156 (15.9423, 15.7321) -> (20.2724, 13.2321)
  line L157 (20.2724, 13.2321) -> (24.6025, 15.7321)
  line L158 (24.6025, 15.7321) -> (24.6025, 20.7321)
  line L159 (24.6025, 20.7321) -> (20.2724, 23.2321)
  line L160 (30.9327, 23.2321) -> (26.6025, 20.7321)
  line L161 (26.6025, 20.7321) -> (26.6025, 15.7321)
  line L162 (26.6025, 15.7321) -> (30.9327, 13.2321)
  line L163 (30.9327, 13.2321) -> (35.2628, 15.7321)
  line L164 (35.2628, 15.7321) -> (35.2628, 20.7321)
  line L165 (35.2628, 20.7321) -> (30.9327, 23.2321)
  line L166 (41.5929, 23.2321) -> (37.2628, 20.7321)
  line L167 (37.2628, 20.7321) -> (37.2628, 15.7321)
  line L168 (37.2628, 15.7321) -> (41.5929, 13.2321)
  line L169 (41.5929, 13.2321) -> (45.923, 15.7321)
  line L170 (45.923, 15.7321) -> (45.923, 20.7321)
  line L171 (45.923, 20.7321) -> (41.5929, 23.2321)
  line L172 (52.2532, 23.2321) -> (47.923, 20.7321)
  line L173 (47.923, 20.7321) -> (47.923, 15.7321)
  line L174 (47.923, 15.7321) -> (52.2532, 13.2321)
  line L175 (52.2532, 13.2321) -> (56.5833, 15.7321)
  line L176 (56.5833, 15.7321) -> (56.5833, 20.7321)
  line L177 (56.5833, 20.7321) -> (52.2532, 23.2321)
  line L178 (62.9134, 23.2321) -> (58.5833, 20.7321)
  line L179 (58.5833, 20.7321) -> (58.5833, 15.7321)
  line L180 (58.5833, 15.7321) -> (62.9134, 13.2321)
  line L181 (62.9134, 13.2321) -> (67.2436, 15.7321)
  line L182 (67.2436, 15.7321) -> (67.2436, 20.7321)
  line L183 (67.2436, 20.7321) -> (62.9134, 23.2321)
  line L184 (73.5737, 23.2321) -> (69.2436, 20.7321)
  line L185 (69.2436, 20.7321) -> (69.2436, 15.7321)
  line L186 (69.2436, 15.7321) -> (73.5737, 13.2321)
  line L187 (73.5737, 13.2321) -> (77.9038, 15.7321)
  line L188 (77.9038, 15.7321) -> (77.9038, 20.7321)
  line L189 (77.9038, 20.7321) -> (73.5737, 23.2321)
  line L190 (-81, 32.4641) -> (-85.3301, 29.9641)
  line L191 (-85.3301, 29.9641) -> (-85.3301, 24.9641)
  line L192 (-85.3301, 24.9641) -> (-81, 22.4641)
  line L193 (-81, 22.4641) -> (-76.6699, 24.9641)
  line L194 (-76.6699, 24.9641) -> (-76.6699, 29.9641)
  line L195 (-76.6699, 29.9641) -> (-81, 32.4641)
  line L196 (-70.3397, 32.4641) -> (-74.6699, 29.9641)
  line L197 (-74.6699, 29.9641) -> (-74.6699, 24.9641)
  line L198 (-74.6699, 24.9641) -> (-70.3397, 22.4641)
  line L199 (-70.3397, 22.4641) -> (-66.0096, 24.9641)
  line L200 (-66.0096, 24.9641) -> (-66.0096, 29.9641)
  line L201 (-66.0096, 29.9641) -> (-70.3397, 32.4641)
  line L202 (-59.6795, 32.4641) -> (-64.0096, 29.9641)
  line L203 (-64.0096, 29.9641) -> (-64.0096, 24.9641)
  line L204 (-64.0096, 24.9641) -> (-59.6795, 22.4641)
  line L205 (-59.6795, 22.4641) -> (-55.3494, 24.9641)
  line L206 (-55.3494, 24.9641) -> (-55.3494, 29.9641)
  line L207 (-55.3494, 29.9641) -> (-59.6795, 32.4641)
  line L208 (-49.0192, 32.4641) -> (-53.3494, 29.9641)
  line L209 (-53.3494, 29.9641) -> (-53.3494, 24.9641)
  line L210 (-53.3494, 24.9641) -> (-49.0192, 22.4641)
  line L211 (-49.0192, 22.4641) -> (-44.6891, 24.9641)
  line L212 (-44.6891, 24.9641) -> (-44.6891, 29.9641)
  line L213 (-44.6891, 29.9641) -> (-49.0192, 32.4641)
  line L214 (-38.359, 32.4641) -> (-42.6891, 29.9641)
  line L215 (-42.6891, 29.9641) -> (-42.6891, 24.9641)
  line L216 (-42.6891, 24.9641) -> (-38.359, 22.4641)
  line L217 (-38.359, 22.4641) -> (-34.0289, 24.9641)
  line L218 (-34.0289, 24.9641) -> (-34.0289, 29.9641)
  line L219 (-34.0289, 29.9641) -> (-38.359, 32.4641)
  line L220 (-27.6987, 32.4641) -> (-32.0289, 29.9641)
  line L221 (-32.0289, 29.9641) -> (-32.0289, 24.9641)
  line L222 (-32.0289, 24.9641) -> (-27.6987, 22.4641)
  line L223 (-27.6987, 22.4641) -> (-23.3686, 24.9641)
  line L224 (-23.3686, 24.9641) -> (-23.3686, 29.9641)
  line L225 (-23.3686, 29.9641) -> (-27.6987, 32.4641)
  line L226 (-17.0385, 32.4641) -> (-21.3686, 29.9641)
  line L227 (-21.3686, 29.9641) -> (-21.3686, 24.9641)
  line L228 (-21.3686, 24.9641) -> (-17.0385, 22.4641)
  line L229 (-17.0385, 22.4641) -> (-12.7083, 24.9641)
  line L230 (-12.7083, 24.9641) -> (-12.7083, 29.9641)
  line L231 (-12.7083, 29.9641) -> (-17.0385, 32.4641)
  line L232 (-6.3782, 32.4641) -> (-10.7083, 29.9641)
  line L233 (-10.7083, 29.9641) -> (-10.7083, 24.9641)
  line L234 (-10.7083, 24.9641) -> (-6.3782, 22.4641)
  line L235 (-6.3782, 22.4641) -> (-2.0481, 24.9641)
  line L236 (-2.0481, 24.9641) -> (-2.0481, 29.9641)
  line L237 (-2.0481, 29.9641) -> (-6.3782, 32.4641)
  line L238 (4.282, 32.4641) -> (-0.0481, 29.9641)
  line L239 (-0.0481, 29.9641) -> (-0.0481, 24.9641)
  line L240 (-0.0481, 24.9641) -> (4.282, 22.4641)
  line L241 (4.282, 22.4641) -> (8.6122, 24.9641)
  line L242 (8.6122, 24.9641) -> (8.6122, 29.9641)
  line L243 (8.6122, 29.9641) -> (4.282, 32.4641)
  line L244 (14.9423, 32.4641) -> (10.6122, 29.9641)
  line L245 (10.6122, 29.9641) -> (10.6122, 24.9641)
  line L246 (10.6122, 24.9641) -> (14.9423, 22.4641)
  line L247 (14.9423, 22.4641) -> (19.2724, 24.9641)
  line L248 (19.2724, 24.9641) -> (19.2724, 29.9641)
  line L249 (19.2724, 29.9641) -> (14.9423, 32.4641)
  line L250 (25.6025, 32.4641) -> (21.2724, 29.9641)
  line L251 (21.2724, 29.9641) -> (21.2724, 24.9641)
  line L252 (21.2724, 24.9641) -> (25.6025, 22.4641)
  line L253 (25.6025, 22.4641) -> (29.9327, 24.9641)
  line L254 (29.9327, 24.9641) -> (29.9327, 29.9641)
  line L255 (29.9327, 29.9641) -> (25.6025, 32.4641)
  line L256 (36.2628, 32.4641) -> (31.9327, 29.9641)
  line L257 (31.9327, 29.9641) -> (31.9327, 24.9641)
  line L258 (31.9327, 24.9641) -> (36.2628, 22.4641)
  line L259 (36.2628, 22.4641) -> (40.5929, 24.9641)
  line L260 (40.5929, 24.9641) -> (40.5929, 29.9641)
  line L261 (40.5929, 29.9641) -> (36.2628, 32.4641)
  line L262 (46.923, 32.4641) -> (42.5929, 29.9641)
  line L263 (42.5929, 29.9641) -> (42.5929, 24.9641)
  line L264 (42.5929, 24.9641) -> (46.923, 22.4641)
  line L265 (46.923, 22.4641) -> (51.2532, 24.9641)
  line L266 (51.2532, 24.9641) -> (51.2532, 29.9641)
  line L267 (51.2532, 29.9641) -> (46.923, 32.4641)
  line L268 (57.5833, 32.4641) -> (53.2532, 29.9641)
  line L269 (53.2532, 29.9641) -> (53.2532, 24.9641)
  line L270 (53.2532, 24.9641) -> (57.5833, 22.4641)
  line L271 (57.5833, 22.4641) -> (61.9134, 24.9641)
  line L272 (61.9134, 24.9641) -> (61.9134, 29.9641)
  line L273 (61.9134, 29.9641) -> (57.5833, 32.4641)
  line L274 (68.2436, 32.4641) -> (63.9134, 29.9641)
  line L275 (63.9134, 29.9641) -> (63.9134, 24.9641)
  line L276 (63.9134, 24.9641) -> (68.2436, 22.4641)
  line L277 (68.2436, 22.4641) -> (72.5737, 24.9641)
  line L278 (72.5737, 24.9641) -> (72.5737, 29.9641)
  line L279 (72.5737, 29.9641) -> (68.2436, 32.4641)
  line L280 (78.9038, 32.4641) -> (74.5737, 29.9641)
  line L281 (74.5737, 29.9641) -> (74.5737, 24.9641)
  line L282 (74.5737, 24.9641) -> (78.9038, 22.4641)
  line L283 (78.9038, 22.4641) -> (83.2339, 24.9641)
  line L284 (83.2339, 24.9641) -> (83.2339, 29.9641)
  line L285 (83.2339, 29.9641) -> (78.9038, 32.4641)
  line L286 (-75.6699, 41.6962) -> (-80, 39.1962)
  line L287 (-80, 39.1962) -> (-80, 34.1962)
  line L288 (-80, 34.1962) -> (-75.6699, 31.6962)
  line L289 (-75.6699, 31.6962) -> (-71.3397, 34.1962)
  line L290 (-71.3397, 34.1962) -> (-71.3397, 39.1962)
  line L291 (-71.3397, 39.1962) -> (-75.6699, 41.6962)
  line L292 (-65.0096, 41.6962) -> (-69.3397, 39.1962)
  line L293 (-69.3397, 39.1962) -> (-69.3397, 34.1962)
  line L294 (-69.3397, 34.1962) -> (-65.0096, 31.6962)
  line L295 (-65.0096, 31.6962) -> (-60.6795, 34.1962)
  line L296 (-60.6795, 34.1962) -> (-60.6795, 39.1962)
  line L297 (-60.6795, 39.1962) -> (-65.0096, 41.6962)
  line L298 (-54.3494, 41.6962) -> (-58.6795, 39.1962)
  line L299 (-58.6795, 39.1962) -> (-58.6795, 34.1962)
  line L300 (-58.6795, 34.1962) -> (-54.3494, 31.6962)
  line L301 (-54.3494, 31.6962) -> (-50.0192, 34.1962)
  line L302 (-50.0192, 34.1962) -> (-50.0192, 39.1962)
  line L303 (-50.0192, 39.1962) -> (-54.3494, 41.6962)
  line L304 (-43.6891, 41.6962) -> (-48.0192, 39.1962)
  line L305 (-48.0192, 39.1962) -> (-48.0192, 34.1962)
  line L306 (-48.0192, 34.1962) -> (-43.6891, 31.6962)
  line L307 (-43.6891, 31.6962) -> (-39.359, 34.1962)
  line L308 (-39.359, 34.1962) -> (-39.359, 39.1962)
  line L309 (-39.359, 39.1962) -> (-43.6891, 41.6962)
  line L310 (-33.0289, 41.6962) -> (-37.359, 39.1962)
  line L311 (-37.359, 39.1962) -> (-37.359, 34.1962)
  line L312 (-37.359, 34.1962) -> (-33.0289, 31.6962)
  line L313 (-33.0289, 31.6962) -> (-28.6987, 34.1962)
  line L314 (-28.6987, 34.1962) -> (-28.6987, 39.1962)
  line L315 (-28.6987, 39.1962) -> (-33.0289, 41.6962)
  line L316 (-22.3686, 41.6962) -> (-26.6987, 39.1962)
  line L317 (-26.6987, 39.1962) -> (-26.6987, 34.1962)
  line L318 (-26.6987, 34.1962) -> (-22.3686, 31.6962)
  line L319 (-22.3686, 31.6962) -> (-18.0385, 34.1962)
  line L320 (-18.0385, 34.1962) -> (-18.0385, 39.1962)
  line L321 (-18.0385, 39.1962) -> (-22.3686, 41.6962)
  line L322 (-11.7083, 41.6962) -> (-16.0385, 39.1962)
  line L323 (-16.0385, 39.1962) -> (-16.0385, 34.1962)
  line L324 (-16.0385, 34.1962) -> (-11.7083, 31.6962)
  line L325 (-11.7083, 31.6962) -> (-7.3782, 34.1962)
  line L326 (-7.3782, 34.1962) -> (-7.3782, 39.1962)
  line L327 (-7.3782, 39.1962) -> (-11.7083, 41.6962)
  line L328 (-1.0481, 41.6962) -> (-5.3782, 39.1962)
  line L329 (-5.3782, 39.1962) -> (-5.3782, 34.1962)
  line L330 (-5.3782, 34.1962) -> (-1.0481, 31.6962)
  line L331 (-1.0481, 31.6962) -> (3.282, 34.1962)
  line L332 (3.282, 34.1962) -> (3.282, 39.1962)
  line L333 (3.282, 39.1962) -> (-1.0481, 41.6962)
  line L334 (9.6122, 41.6962) -> (5.282, 39.1962)
  line L335 (5.282, 39.1962) -> (5.282, 34.1962)
  line L336 (5.282, 34.1962) -> (9.6122, 31.6962)
  line L337 (9.6122, 31.6962) -> (13.9423, 34.1962)
  line L338 (13.9423, 34.1962) -> (13.9423, 39.1962)
  line L339 (13.9423, 39.1962) -> (9.6122, 41.6962)
  line L340 (20.2724, 41.6962) -> (15.9423, 39.1962)
  line L341 (15.9423, 39.1962) -> (15.9423, 34.1962)
  line L342 (15.9423, 34.1962) -> (20.2724, 31.6962)
  line L343 (20.2724, 31.6962) -> (24.6025, 34.1962)
  line L344 (24.6025, 34.1962) -> (24.6025, 39.1962)
  line L345 (24.6025, 39.1962) -> (20.2724, 41.6962)
  line L346 (30.9327, 41.6962) -> (26.6025, 39.1962)
  line L347 (26.6025, 39.1962) -> (26.6025, 34.1962)
  line L348 (26.6025, 34.1962) -> (30.9327, 31.6962)
  line L349 (30.9327, 31.6962) -> (35.2628, 34.1962)
  line L350 (35.2628, 34.1962) -> (35.2628, 39.1962)
  line L351 (35.2628, 39.1962) -> (30.9327, 41.6962)
  line L352 (41.5929, 41.6962) -> (37.2628, 39.1962)
  line L353 (37.2628, 39.1962) -> (37.2628, 34.1962)
  line L354 (37.2628, 34.1962) -> (41.5929, 31.6962)
  line L355 (41.5929, 31.6962) -> (45.923, 34.1962)
  line L356 (45.923, 34.1962) -> (45.923, 39.1962)
  line L357 (45.923, 39.1962) -> (41.5929, 41.6962)
  line L358 (52.2532, 41.6962) -> (47.923, 39.1962)
  line L359 (47.923, 39.1962) -> (47.923, 34.1962)
  line L360 (47.923, 34.1962) -> (52.2532, 31.6962)
  line L361 (52.2532, 31.6962) -> (56.5833, 34.1962)
  line L362 (56.5833, 34.1962) -> (56.5833, 39.1962)
  line L363 (56.5833, 39.1962) -> (52.2532, 41.6962)
  line L364 (62.9134, 41.6962) -> (58.5833, 39.1962)
  line L365 (58.5833, 39.1962) -> (58.5833, 34.1962)
  line L366 (58.5833, 34.1962) -> (62.9134, 31.6962)
  line L367 (62.9134, 31.6962) -> (67.2436, 34.1962)
  line L368 (67.2436, 34.1962) -> (67.2436, 39.1962)
  line L369 (67.2436, 39.1962) -> (62.9134, 41.6962)
  line L370 (73.5737, 41.6962) -> (69.2436, 39.1962)
  line L371 (69.2436, 39.1962) -> (69.2436, 34.1962)
  line L372 (69.2436, 34.1962) -> (73.5737, 31.6962)
  line L373 (73.5737, 31.6962) -> (77.9038, 34.1962)
  line L374 (77.9038, 34.1962) -> (77.9038, 39.1962)
  line L375 (77.9038, 39.1962) -> (73.5737, 41.6962)
extrude "cut_hex_drawer_right" cut sketch "草图70" against normal blind 3 contours L4 L5 L6 L7 L8 L9 | L10 L11 L12 L13 L14 L15 | L16 L17 L18 L19 L20 L21 | L22 L23 L24 L25 L26 L27 | L28 L29 L30 L31 L32 L33 | L34 L35 L36 L37 L38 L39 | L40 L41 L42 L43 L44 L45 | L46 L47 L48 L49 L50 L51 | L52 L53 L54 L55 L56 L57 | L58 L59 L60 L61 L62 L63 | L64 L65 L66 L67 L68 L69 | L70 L71 L72 L73 L74 L75 | L76 L77 L78 L79 L80 L81 | L82 L83 L84 L85 L86 L87 | L88 L89 L90 L91 L92 L93 | L94 L95 L96 L97 L98 L99 | L100 L101 L102 L103 L104 L105 | L106 L107 L108 L109 L110 L111 | L112 L113 L114 L115 L116 L117 | L118 L119 L120 L121 L122 L123 | L124 L125 L126 L127 L128 L129 | L130 L131 L132 L133 L134 L135 | L136 L137 L138 L139 L140 L141 | L142 L143 L144 L145 L146 L147 | L148 L149 L150 L151 L152 L153 | L154 L155 L156 L157 L158 L159 | L160 L161 L162 L163 L164 L165 | L166 L167 L168 L169 L170 L171 | L172 L173 L174 L175 L176 L177 | L178 L179 L180 L181 L182 L183 | L184 L185 L186 L187 L188 L189 | L190 L191 L192 L193 L194 L195 | L196 L197 L198 L199 L200 L201 | L202 L203 L204 L205 L206 L207 | L208 L209 L210 L211 L212 L213 | L214 L215 L216 L217 L218 L219 | L220 L221 L222 L223 L224 L225 | L226 L227 L228 L229 L230 L231 | L232 L233 L234 L235 L236 L237 | L238 L239 L240 L241 L242 L243 | L244 L245 L246 L247 L248 L249 | L250 L251 L252 L253 L254 L255 | L256 L257 L258 L259 L260 L261 | L262 L263 L264 L265 L266 L267 | L268 L269 L270 L271 L272 L273 | L274 L275 L276 L277 L278 L279 | L280 L281 L282 L283 L284 L285 | L286 L287 L288 L289 L290 L291 | L292 L293 L294 L295 L296 L297 | L298 L299 L300 L301 L302 L303 | L304 L305 L306 L307 L308 L309 | L310 L311 L312 L313 L314 L315 | L316 L317 L318 L319 L320 L321 | L322 L323 L324 L325 L326 L327 | L328 L329 L330 L331 L332 L333 | L334 L335 L336 L337 L338 L339 | L340 L341 L342 L343 L344 L345 | L346 L347 L348 L349 L350 L351 | L352 L353 L354 L355 L356 L357 | L358 L359 L360 L361 L362 L363 | L364 L365 L366 L367 L368 L369 | L370 L371 L372 L373 L374 L375